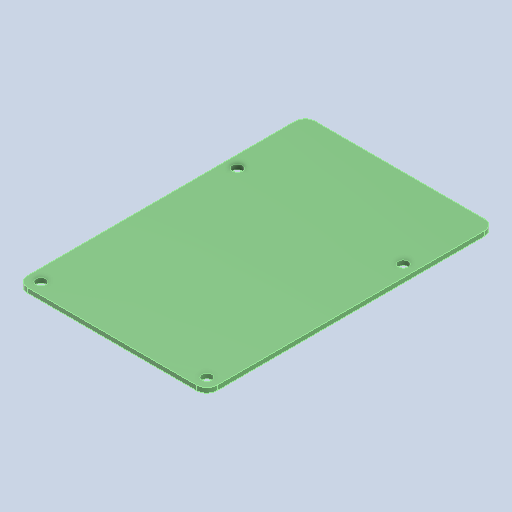
# Autodesk Inventor part: Raspberry Pi
Saved by Autodesk Inventor 2022.3 (Build 263350030, 350C)
## iProperties
Created: 2024-06-08
Part Number: Raspberry Pi
Material: Generic
Document SubType Name: Modeling
Designer: david
Density: 1 g/cm^3
Appearance: Smooth - Dark Forest Green
Description: Controller
Mass: 6.6136 g
Surface Area: 98.8837 cm^2
Volume: 6.6136 cm^3
Author: david
Autodesk Inventor part; units mm, degrees
ref_plane "YZ Plane" through (0, 0, 0) normal (1, 0, 0) x (0, 1, 0)
ref_plane "XZ Plane" through (0, 0, 0) normal (0, 1, 0) x (-1, 0, 0)
ref_plane "XY Plane" through (0, 0, 0) normal (0, 0, 1) x (1, 0, 0)
sketch "Sketch1" plane through (0, 0, 0) normal (0, 1, 0) x (-1, 0, 0)
  line L0 (28, -85) -> (-28, -85)
  line L1 (-28, -85) -> (-28, 0)
  line L2 (-28, 0) -> (28, 0)
  line L3 (28, 0) -> (28, -85)
  point P0 (0, 0)
  point P1 (0, 0)
  dimension "d0" = 85
  dimension "d1" = 56
  constraints: 8 end point, 2 coincident, 2 parallel, 1 horizontal, 1 midpoint, 1 perpendicular
  measures "d0" distance of L0.end L1.end
  measures "d1" distance of L0.start L0.end
extrude "Extrusion1" add sketch "Sketch1" along normal blind 1.4
fillet "Fillet1" radius 3 4 edges at (-28, 0.7, 0) (28, 0.7, 0) (28, 0.7, -85) (-28, 0.7, -85)
sketch "Sketch2" plane through (0, 1.4, 0) normal (0, 1, 0) x (1, 0, 0)
  line L0 (-24.5, 61.5) -> (24.5, 61.5) construction
  line L1 (24.5, 61.5) -> (24.5, 3.5) construction
  line L2 (24.5, 3.5) -> (-24.5, 3.5) construction
  line L3 (-24.5, 3.5) -> (-24.5, 61.5) construction
  line L4 (-28, 82) -> (-28, 3) construction
  line L5 (-25, 0) -> (25, 0) construction
  point P0 (0, 0)
  dimension "d5" = 49
  dimension "d6" = 58
  dimension "d7" = 3.5
  dimension "d8" = 3.5
  constraints: 8 end point, 4 coincident, 2 parallel, 1 horizontal, 1 perpendicular
  measures "d5" distance of L1.end L2.end
  measures "d6" distance of L2.end L0.start
  measures "d7" distance between parallel lines of L3 L4
  measures "d8" distance from line of L5 L2.end
hole "Hole1" at (-24.5, 1.4, -61.5) at (24.5, 1.4, -61.5) at (24.5, 1.4, -3.5) at (-24.5, 1.4, -3.5) direction (0, -1, 0) diameter 3 depth 6
body "Solid1"
